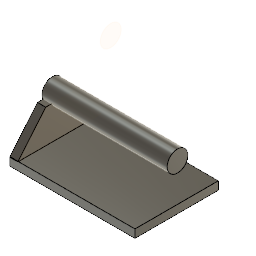
Desktrunk-Clip (Autodesk Fusion 360 design; units mm, degrees)
Autodesk Fusion 360 part; units mm, degrees
sketch "Sketch1" plane through (0, 0, 0) normal (1, 0, 0) x (0, 1, 0)
  line L0 (-5, 6) -> (11.1286, 6)
  line L1 (11.1286, 6) -> (11.1286, -7.5034)
  line L2 (11.1286, -7.5034) -> (-5, -7.5034)
  line L3 (-5, -7.5034) -> (-5, 6)
  constraint horizontal L0
  constraint vertical L1
  constraint horizontal L2
  constraint vertical L3
sketch "Sketch2" plane through (0, 0, 0) normal (1, 0, 0) x (0, 1, 0)
  line L0 (-28, 22) -> (-16, 22)
  line L1 (-16, 22) -> (-16, 10.6443)
  line L2 (-16, 10.6443) -> (-36, 10.6443)
  line L3 (-36, 10.6443) -> (-28, 22)
  constraint horizontal L0
  constraint perpendicular L0 L1
  constraint perpendicular L1 L2
sketch "Sketch3" plane through (0, 0, 0) normal (0, 0, 1) x (1, 0, 0)
  circle A0 centre (-31.5, 17.5) radius 1.5811
sketch "Sketch4" plane through (0, 0, 0) normal (0, 0, 1) x (1, 0, 0)
  line L0 (-20, 25) -> (-5, 25)
  line L1 (-5, 25) -> (-5, 5)
  line L2 (-5, 5) -> (-20, 5)
  line L3 (-20, 5) -> (-20, 25)
  constraint horizontal L0
  constraint vertical L1
  constraint horizontal L2
  constraint vertical L3
sketch "Sketch5" plane through (0, 0, 2.8539) normal (0, 0, 1) x (-1, 0, 0)
  line L0 (20, -5) -> (5, -5)
  line L1 (5, -5) -> (5, -25)
  line L2 (5, -25) -> (20, -25)
  line L3 (20, -25) -> (20, -5)
  line L4 (13.5, -20) -> (10.5, -20)
  arc A0 (10.5, -18.5) -> (10.5, -20) centre (10.5, -19.25) ccw
  line L5 (10.5, -18.5) -> (13.5, -18.5)
  arc A1 (13.5, -20) -> (13.5, -18.5) centre (13.5, -19.25) ccw
  constraint horizontal L4
  constraint tangent L4 A0
  constraint tangent A0 L5
  constraint parallel L4 L5
  constraint tangent L5 A1
  constraint tangent L4 A1
sketch "Sketch6" plane through (0, 0, 2.8539) normal (0, 0, 1) x (-1, 0, 0)
  line L0 (13.5, -20) -> (10.5, -20)
  arc A0 (10.5, -18.5) -> (10.5, -20) centre (10.5, -19.25) ccw
  line L1 (10.5, -18.5) -> (13.5, -18.5)
  arc A1 (13.5, -20) -> (13.5, -18.5) centre (13.5, -19.25) ccw
  line L2 (20, -5) -> (5, -5)
  line L3 (5, -5) -> (5, -25)
  line L4 (5, -25) -> (20, -25)
  line L5 (20, -25) -> (20, -5)
  circle A2 centre (12, -7) radius 1
  dimension "d11" = 2
  measures "d11" diameter of A2
sketch "Sketch7" plane through (0, 0, 0) normal (0, 0, 1) x (1, 0, 0)
  line L0 (-5, 10) -> (-15, 10)
  line L1 (-15, 10) -> (-15, -32)
  line L2 (-15, -32) -> (-5, -32)
  line L3 (-5, -32) -> (-5, 10)
  dimension "d14" = 42
  dimension "d15" = 10
  constraint horizontal L0
  constraint vertical L1
  constraint horizontal L2
  constraint vertical L3
  measures "d14" distance of L0.start L2.end
  measures "d15" distance of L0.start L0.end
sketch "Sketch8" plane through (0, 0, 2) normal (0, 0, 1) x (-1, 0, 0)
  line L0 (5, 32) -> (5, -10)
  line L1 (5, -10) -> (15, -10)
  line L2 (15, -10) -> (15, 32)
  line L3 (15, 32) -> (5, 32)
  circle A0 centre (10, -6.5) radius 1.5
  dimension "d18" = 3
  measures "d18" diameter of A0
sketch "Sketch9" plane through (0, 0, 0) normal (0, 0, 1) x (1, 0, 0)
  line L0 (-15, -32) -> (-5, -32)
  line L1 (-15, 10) -> (-15, -32)
  line L2 (-12, -29) -> (-8, -29)
  line L3 (-8, -26) -> (-12, -26)
  ellipse E0 centre (-12, -27.5) end of major axis (-12, -29) minor radius 0.5003 (-12, -26) -> (-12, -29) ccw
  ellipse E1 centre (-8, -27.5) end of major axis (-8, -29) minor radius 0.5011 (-8, -29) -> (-8, -26) ccw
  constraint horizontal L2
sketch "Sketch10" plane through (0, 0, 0) normal (0, 0, 1) x (1, 0, 0)
  line L0 (-5, 10) -> (-15, 10)
  line L1 (15, -15) -> (35, -15)
  line L2 (15, -15) -> (15, -5)
  line L3 (15, -5) -> (35, -5)
  line L4 (35, -5) -> (35, -15)
  dimension "d27" = 20
  constraint parallel L0 L1
  constraint coincident L1 L2.start
  constraint perpendicular L1 L2
  constraint perpendicular L2 L3
  measures "d27" distance of L1.start L1.end
extrude "Extrude10" add sketch "Sketch10" along normal blind 1 makes body 1
sketch "Sketch11" plane through (0, 0, 0) normal (1, 0, 0) x (0, 1, 0)
  line L0 (-32, 0) -> (10, 0)
  line L1 (-5, 0) -> (-5, 1)
  line L2 (-15, 0) -> (-5, 0)
  line L3 (-5, 0) -> (-7.5, 3)
  line L4 (-7.5, 3) -> (-12.5, 3)
  line L5 (-12.5, 3) -> (-15, 0)
  point P0 (-15, 0)
  point P1 (-15, 0)
  constraint coincident P0 L2.start
  constraint coincident L0 L1.start
  constraint perpendicular L1 L2
  constraint coincident L1.start L2.end
  constraint perpendicular L1 L4
  constraint coincident P1 P0
extrude "Extrude11" add sketch "Sketch11" along normal blind 1 separate body makes body 2
move_body "Move3" bodies 2 to x (1, 0, 0) y (0, 1, 0) z (0, 0, 1) at (4, 0.7682, 0.6402)
sketch "Sketch12" plane through (0, 0, 0) normal (1, 0, 0) x (0, 1, 0)
  circle A0 centre (-2.5, 7.5) radius 1.25
  dimension "d32" = 2.5
  measures "d32" diameter of A0
extrude "Extrude12" add sketch "Sketch12" along normal blind 15 separate body makes body 3
move_face "MoveFace2" by (0, 0, 1) 1 faces at (4.3333, -8.3984, 3.6402) on bodies 2
move_body "Move4" bodies 2 to x (1, 0, 0) y (0, 1, 0) z (0, 0, 1) at (11, -0.3841, 0.3201)
move_body "Move5" bodies 1 to x (1, 0, 0) y (0, 1, 0) z (0, 0, 1) at (0, 0.4, 0)
sketch "Sketch13" plane through (15, 0, 0) normal (1, 0, 0) x (0, 1, 0)
  circle A0 centre (-2.5, 7.5) radius 1.25
move_face "MoveFace3" to x (1, 0, 0) y (0, 1, 0) z (0, 0, 1) at (20, 0, 0) 1 faces at (10, -1.2562, 7.3755) on bodies 3
move_body "Move6" bodies 3 to x (1, 0, 0) y (0, 1, 0) z (0, 0, 1) at (15, -7, -2)
sketch "Sketch14" plane through (16, 0, 0) normal (1, 0, 0) x (0, 1, 0)
  line L0 (-11.2826, 4.9603) -> (-14.6159, 0.9603)
  line L1 (-14.6159, 0.9603) -> (-4.6159, 0.9603)
  line L2 (-4.6159, 0.9603) -> (-7.9492, 4.9603)
  line L3 (-7.9492, 4.9603) -> (-11.2826, 4.9603)
sketch "Sketch15" plane through (0, 0, 0) normal (0, 0, 1) x (1, 0, 0)
  line L0 (15, -14.6) -> (35, -14.6)
  line L1 (30, -3.6592) -> (30, -16.2646)
  line L2 (30, -16.2646) -> (36, -16.2646)
  line L3 (36, -16.2646) -> (36, -3.5)
  line L4 (36, -3.5) -> (30, -3.6592)
  constraint perpendicular L0 L1
  constraint perpendicular L1 L2
  constraint perpendicular L2 L3
extrude "Extrude13" cut sketch "Sketch15" along normal blind 5 bodies 1
